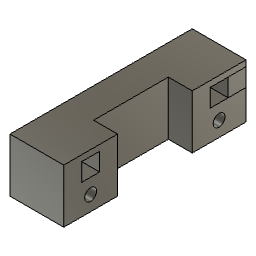
Gancho+Corda (Autodesk Fusion 360 design; units mm, degrees)
Autodesk Fusion 360 part; units mm, degrees
sketch "Esboço6" plane through (0, 0, 0) normal (0, 0, 1) x (1, 0, 0)
  line L0 (75, 0, 10) -> (93, 0, 10)
  line L1 (75, 0, 10) -> (75, 61, 10)
  line L2 (75, 61, 10) -> (93, 61, 10)
  line L3 (93, 18, 10) -> (85, 18, 10)
  line L4 (93, 43, 10) -> (85, 43, 10)
  line L5 (85, 43, 10) -> (85, 18, 10)
  line L6 (93, 18, 10) -> (93, 12, 10)
  line L7 (93, 0, 10) -> (93, 6, 10)
  line L8 (93, 6, 10) -> (77, 6, 10)
  line L9 (75, 61, 10) -> (75, 55, 10)
  line L10 (77, 6, 10) -> (77, 55, 10)
  line L11 (83, 43, 10) -> (83, 12, 10)
  line L12 (83, 12, 10) -> (93, 12, 10)
  line L13 (93, 18, 10) -> (93, 12, 10)
  line L14 (93, 6, 10) -> (93, 0, 10)
  line L15 (83, 43, 10) -> (83, 49, 10)
  line L16 (83, 49, 10) -> (93, 49, 10)
  line L17 (77, 55, 10) -> (93, 55, 10)
  line L18 (93, 43, 10) -> (93, 49, 10)
  line L19 (93, 55, 10) -> (93, 61, 10)
  dimension "d52" = 18
  dimension "d53" = 61
  dimension "d54" = 18
  dimension "d55" = 18
  dimension "d56" = 18
  dimension "d58" = 8
  dimension "d59" = 2
  dimension "d64" = 6
sketch "Esboço7" plane through (0, 0, 0) normal (0, 0, 1) x (1, 0, 0)
  line L0 (75, 61) -> (93, 61)
  line L1 (93, 61) -> (93, 43)
  line L2 (85, 43) -> (85, 18)
  line L3 (85, 18) -> (93, 18)
  line L4 (93, 18) -> (93, 0)
  line L5 (93, 0) -> (75, 0)
  line L6 (75, 0) -> (75, 61)
  line L7 (93, 43) -> (85, 43)
  constraint horizontal L0
  constraint perpendicular L0 L1
  constraint perpendicular L0 L2
  constraint perpendicular L2 L3
  constraint perpendicular L0 L4
  constraint perpendicular L4 L5
  constraint perpendicular L0 L6
  constraint perpendicular L2 L7
sketch "Esboço8" plane through (0, 0, 0) normal (0, 0, 1) x (1, 0, 0)
  line L0 (93, 18) -> (93, 9.7778)
  line L1 (93, 0) -> (93, 9.7778)
  line L2 (93, 0) -> (75, 0)
  line L3 (75, 0) -> (75, 61)
  line L4 (75, 61) -> (93, 61)
  line L5 (93, 18) -> (85, 18)
  line L6 (85, 18) -> (85, 43)
  line L7 (85, 43) -> (93, 43)
  line L8 (93, 54.5) -> (93.0266, 54.5)
  line L9 (93, 49.5) -> (93.0266, 49.5)
  line L10 (93, 43) -> (93, 61)
  constraint vertical L0
  constraint parallel L0 L1
  constraint perpendicular L1 L2
  constraint perpendicular L2 L3
  constraint perpendicular L3 L4
  constraint perpendicular L0 L5
  constraint perpendicular L5 L6
  constraint perpendicular L0 L7
  constraint perpendicular L4 L10
extrude "Extrusão12" add sketch "Esboço7" along normal blind 2
extrude "Extrusão13" add sketch "Esboço8" along normal blind 5 from surface at 2
extrude "Extrusão14" add sketch "Esboço7" along normal blind 3 from surface at 7
ref_plane "Plano de trabalho3" through (0, 0, 11) normal (0, 0, 1) x (1, 0, 0)
extrude "Extrusão15" add sketch "Esboço6" along normal blind 6 contours L0 L1 L2 L7 L8 L9 L10 L14 L17 L19 | L3 L4 L5 L6 L11 L12 L13 L15 L16 L18 in plane through (0, 0, 10) normal (0, 0, 1)
extrude "Extrusão16" add sketch "Esboço7" along normal blind 2 from surface at 16
fillet "Arredondamento7" radius 2 2 edges at (83, 49, 13) (83, 12, 13)
sketch "Esboço14" plane through (93, 0, 0) normal (1, 0, 0) x (0, 1, 0)
  line L0 (0, 18) -> (0, 0)
  line L1 (0, 0) -> (18, 0)
  line L2 (18, 0) -> (18, 18)
  line L3 (18, 18) -> (0, 18)
  line L4 (6, 16) -> (12, 16)
  line L5 (12, 16) -> (12, 10)
  line L6 (12, 10) -> (6, 10)
  line L7 (6, 10) -> (6, 16)
  line L8 (55, 16) -> (49, 16)
  circle A0 centre (9, 5) radius 2
  circle A1 centre (52, 5) radius 2
  dimension "d103" = 4
  dimension "d104" = 4
  constraint horizontal L8
  measures "d103" diameter of A0
  measures "d104" diameter of A1
extrude "Extrusão17" cut sketch "Esboço14" against normal blind 8 contours A1
extrude "Extrusão18" cut sketch "Esboço14" against normal blind 8 contours A0
